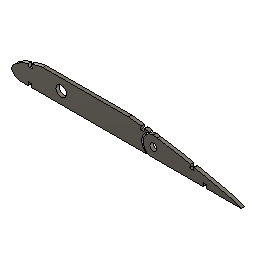
Wing back flap v1 (Autodesk Fusion 360 design; units mm, degrees)
Autodesk Fusion 360 part; units mm, degrees
note: some values were not read from the file. Set by a fixed rule: which sketch regions a step uses.
sketch "Sketch1" plane through (0, 0, 0) normal (0, 0, 1) x (1, 0, 0) in component "Airfoil structure"
  spline S0 degree 5 poles (108.4381, 17.4711) (108.649, 17.4404) (108.9954, 17.3905) (109.2888, 17.35) (109.4947, 17.3216) (110.5176, 17.1554) (112.7992, 16.78) (116.3579, 16.1938) (120.8926, 15.4471) (125.9053, 14.6214) (130.826, 13.8088) (135.1336, 13.0925) (138.4727, 12.5267) (140.7909, 12.1145) (142.442, 11.7905) (143.9925, 11.4539) (145.6494, 11.0874) (147.355, 10.7177) (148.7282, 10.4238) (149.4739, 10.265) knots 0 0 0 0 0 0 0.066667 0.133333 0.2 0.266667 0.333333 0.4 0.466667 0.533333 0.6 0.666667 0.733333 0.8 0.866667 0.933333 1 1 1 1 1 1
  line L0 (104.3157, 18.0708) -> (112.5606, 16.8713)
  line L1 (145.4959, 11.1121) -> (153.4519, 9.4178)
  spline S1 degree 5 poles (152.8506, 9.5306) (153.6754, 9.3537) (155.1958, 9.0286) (157.0885, 8.6275) (158.936, 8.2427) (160.6637, 7.8882) (162.4454, 7.5152) (164.8302, 6.998) (168.0436, 6.2836) (171.9512, 5.3995) (176.2203, 4.4165) (180.4192, 3.4262) (184.1363, 2.5128) (187.0894, 1.7283) (189.2467, 1.0647) (190.9412, 0.4271) (192.3181, -0.1661) (193.5665, -0.7107) (194.5238, -1.1255) (195.0337, -1.3459) knots 0 0 0 0 0 0 0.066667 0.133333 0.2 0.266667 0.333333 0.4 0.466667 0.533333 0.6 0.666667 0.733333 0.8 0.866667 0.933333 1 1 1 1 1 1
  line L2 (148.4907, 10.4656) -> (157.2105, 8.5955)
  line L3 (191.9852, -0.0284) -> (198.0822, -2.6634)
  circle A0 centre (33.1388, 9.1296) radius 4.765
  circle A1 centre (116.1615, 7.0362) radius 3.175
  spline S2 degree 5 poles (-3.081, -1.3459) (-3.6016, -1.2531) (-4.5413, -1.0758) (-5.6462, -0.8349) (-6.5938, -0.5667) (-7.329, -0.2952) (-8.0514, 0.0089) (-9.0194, 0.5708) (-10.0684, 1.7874) (-10.9642, 3.2519) (-11.5103, 4.4866) (-11.5777, 5.0951) (-11.407, 5.643) (-11.0112, 6.6068) (-10.1307, 7.993) (-8.6022, 9.6432) (-6.4034, 11.2721) (-4.1965, 12.5716) (-2.7349, 13.4061) (-1.8316, 13.8946) (-1.0216, 14.2664) (0.0955, 14.6934) (1.459, 15.1917) (2.6392, 15.6173) (3.2971, 15.8534) knots 0 0 0 0 0 0 0.05 0.1 0.15 0.2 0.25 0.3 0.35 0.4 0.45 0.5 0.55 0.6 0.65 0.7 0.75 0.8 0.85 0.9 0.95 1 1 1 1 1 1
  line L4 (0.5703, -1.9966) -> (-6.7323, -0.6952)
  line L5 (-0.0118, 14.6656) -> (6.606, 17.0412)
  line L6 (-8.4792, 9.8153) -> (-3.9569, 12.8132)
  line L7 (-11.5034, 4.2257) -> (-11.5345, 5.6935)
  line L8 (-7.2174, -0.5359) -> (-9.7443, 1.1286)
  line L9 (16.5688, 19.3646) -> (93.5688, 19.3646)
  spline S3 degree 5 poles (93.5688, 19.3646) (93.8188, 19.3387) (94.2829, 19.2905) (94.8714, 19.229) (95.4658, 19.1659) (96.0263, 19.1049) (96.567, 19.0445) (97.2368, 18.9678) (98.1315, 18.8622) (99.3129, 18.7173) (100.8213, 18.5245) (102.3116, 18.3263) (103.5971, 18.1504) (104.5298, 18.0208) (105.015, 17.9529) knots 0 0 0 0 0 0 0.1 0.2 0.3 0.4 0.5 0.6 0.7 0.8 0.9 1 1 1 1 1 1
  line L10 (92.266, 19.4996) -> (94.8715, 19.2297)
  line L11 (103.6445, 18.1447) -> (106.3855, 17.761)
  spline S4 degree 5 poles (6.5765, 16.943) (6.9079, 17.0449) (7.5374, 17.2364) (8.3817, 17.4868) (9.3156, 17.7508) (10.2084, 17.9865) (10.8922, 18.156) (11.4504, 18.29) (11.9864, 18.4184) (12.6265, 18.5675) (13.504, 18.76) (14.4962, 18.9637) (15.447, 19.1503) (16.1786, 19.2906) (16.5688, 19.3646) knots 0 0 0 0 0 0 0.1 0.2 0.3 0.4 0.5 0.6 0.7 0.8 0.9 1 1 1 1 1 1
  line L12 (5.4107, 16.5846) -> (7.7424, 17.3015)
  line L13 (15.2328, 19.111) -> (17.9048, 19.6183)
  line L14 (152.4045, 9.626) -> (152.8506, 9.5306)
  line L15 (107.9857, 17.5357) -> (108.4381, 17.4711)
  line L16 (6.1441, 16.7993) -> (6.5765, 16.943)
  line L17 (128.8588, -1.3459) -> (132.3138, -1.3459)
  line L18 (149.4739, 10.265) -> (148.8437, 7.3202)
  line L19 (148.8437, 7.3202) -> (151.7767, 6.6924)
  line L20 (151.7767, 6.6924) -> (152.4045, 9.626)
  line L21 (105.015, 17.9529) -> (104.5907, 14.9843)
  line L22 (104.5907, 14.9843) -> (107.5603, 14.5598)
  line L23 (107.5603, 14.5598) -> (107.9857, 17.5357)
  line L24 (3.2971, 15.8534) -> (4.243, 13.0064)
  line L25 (4.243, 13.0064) -> (7.09, 13.9524)
  line L26 (7.09, 13.9524) -> (6.1441, 16.7993)
  line L27 (160.8934, -1.3459) -> (160.8934, 1.6536)
  line L28 (160.8934, 1.6536) -> (163.8934, 1.6536)
  line L29 (163.8934, 1.6536) -> (163.8934, -1.3459)
  line L30 (132.3138, -1.3459) -> (160.8934, -1.3459)
  line L31 (163.8934, -1.3459) -> (195.0337, -1.3459)
  line L32 (3.4513, -1.3459) -> (3.4513, 1.6536)
  line L33 (3.4513, 1.6536) -> (6.4513, 1.6536)
  line L34 (6.4513, 1.6536) -> (6.4513, -1.3459)
  line L35 (-3.081, -1.3459) -> (3.4513, -1.3459)
  line L36 (6.4513, -1.3459) -> (128.8588, -1.3459)
  circle A2 centre (116.1615, 7.0362) radius 9.25
  circle A3 centre (116.1615, 7.0362) radius 10.5
  point P0 (-8.4808, 0.2964)
  point P1 (-11.5189, 4.9596)
  point P2 (-6.2181, 11.3142)
  point P3 (11.4183, 18.2822)
  point P4 (96.5722, 19.0435)
  point P5 (109.7252, 17.2828)
  point P6 (137.8534, 12.6279)
  point P7 (163.7248, 7.2358)
  point P8 (186.791, 1.7868)
  dimension "d38" = 77
  dimension "d53" = 9.53
  dimension "d54" = 6.35
  dimension "d60" = 83.0226
  dimension "d64" = 18.5
  dimension "d65" = 21
  constraint midpoint S0.start L0
  constraint midpoint S0.end L1
  constraint midpoint S1.start L2
  constraint midpoint S1.end L3
  constraint midpoint S2.start L4
  constraint midpoint S2.end L5
  constraint midpoint P2 L6
  constraint midpoint P1 L7
  constraint midpoint P0 L8
  constraint horizontal L9
  constraint midpoint L9.end L10
  constraint midpoint S3.end L11
  constraint midpoint S4.start L12
  constraint midpoint L9.start L13
  constraint parallel L30 L35
  constraint collinear L30 L35
  constraint horizontal L35
  constraint parallel L17 L30
  constraint perpendicular L14 L18
  constraint perpendicular L18 L19
  constraint perpendicular L14 L20
  constraint perpendicular L15 L21
  constraint perpendicular L21 L22
  constraint perpendicular L15 L23
  constraint perpendicular L16 L24
  constraint perpendicular L24 L25
  constraint perpendicular L16 L26
  constraint perpendicular L27 L30
  constraint perpendicular L27 L28
  constraint perpendicular L28 L29
  constraint collinear L30 L31
  constraint perpendicular L32 L35
  constraint perpendicular L32 L33
  constraint coincident L34.end L35
  constraint perpendicular L34 L35
  constraint collinear L35 L36
  constraint concentric A1 A2
  constraint concentric A1 A3
  measures "d38" distance of L9.start L9.end
  measures "d53" diameter of A0
  measures "d54" diameter of A1
  measures "d60" horizontal distance of A0.centre A1.centre
  measures "d64" diameter of A2
  measures "d65" diameter of A3
extrude "Extrude1" add sketch "Sketch1" along normal blind 3 contours S0 L0 S2 L9 S3 L10 L11 S4 L15 L16 L21 L22 L23 L24 L25 L26 L32 L33 L34 L35 L36 A3 | S0 L36 A2 | S0 L36 A2 A3 | S0 S1 L2 L3 L14 L17 L18 L19 L20 L27 L28 L29 L30 L31 L36 A3 picked at (123.1311, 14.2971) makes body 1 at (79.1074, 9.933, 0) makes body 2 at (134.8814, 8.0108, 0) in component "Airfoil structure"
sketch "Sketch3" plane through (0, 0, 0) normal (0, 0, 1) x (1, 0, 0)
component "Airfoil structure" placed x (1, 0, 0) y (0, 1, 0) z (0, 0, 1) at (0, 0, 0)
